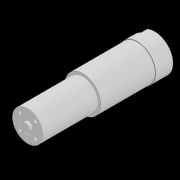
# Autodesk Inventor part: ShoulderServo
Saved by Autodesk Inventor 2020 (Build 240168000, 168)
## iProperties
Created: 2021-01-27
Part Number: ShoulderServo
Material: Generic
Document SubType Name: Modeling
Designer: valer
Density: 1 g/cm^3
Appearance: Default
Author: valer
Autodesk Inventor part; units mm, degrees
ref_plane "YZ Plane" through (0, 0, 0) normal (1, 0, 0) x (0, 1, 0)
ref_plane "XZ Plane" through (0, 0, 0) normal (0, 1, 0) x (-1, 0, 0)
ref_plane "XY Plane" through (0, 0, 0) normal (0, 0, 1) x (1, 0, 0)
sketch "Base" plane through (0, 0, 0) normal (0, 0, 1) x (1, 0, 0)
  circle A0 centre (0, 0) radius 18.75
  dimension "d0" = 37.5
  constraints: 1 centre point, 1 coincident
  measures "d0" diameter of A0
extrude "BaseFeature" add sketch "Base" along normal blind 57
sketch "Sketch2" plane through (0, 0, 0) normal (0, 0, -1) x (-1, 0, 0)
  circle A0 centre (0, 0) radius 18.75 projected
  circle A1 centre (0, 0) radius 19.25
  dimension "d3" = 0.5
  constraints: 1 centre point, 1 coincident
  measures "d3" radial gap between concentric circles of A1 A0
extrude "BottomFeature" add sketch "Sketch2" along normal blind 18.2 contours A0 | A1
sketch "Panel" plane through (0, 0, -18.2) normal (0, 0, -1) x (-1, 0, 0)
  circle A0 centre (0, 0) radius 19.25 projected
  line L0 (7.75, 17.621) -> (7.75, -17.621)
  circle A1 centre (0, 0) radius 18.75 construction
  line L1 (0, 0) -> (-19.25, 0) construction
  circle A2 centre (0, 0) radius 19.25 projected
  line L2 (7.75, 17.621) -> (19.25, 17.621)
  line L3 (19.25, 17.621) -> (19.25, -17.621)
  line L4 (19.25, -17.621) -> (7.75, -17.621)
  line L5 (7.75, -17.621) -> (7.75, 17.621)
  dimension "d6" = 27
  constraints: 12 end point, 3 point on circle, 2 horizontal, 2 parallel, 1 perpendicular, 1 point on line, 1 tangent, 1 vertical
  measures "d6" distance from line of L1.end L0
extrude "PanelFeature" cut sketch "Panel" against normal blind 6.5 contours A0 L0 picked at (11.5833, 0)
sketch "Gearbox" plane through (0, 0, 57) normal (0, 0, 1) x (1, 0, 0)
  circle A0 centre (0, 0) radius 16
  dimension "d9" = 32
  constraints: 1 centre point, 1 coincident
  measures "d9" diameter of A0
extrude "GearboxFeature" add sketch "Gearbox" along normal blind 57.8
sketch "Shaft" plane through (0, 0, 114.8) normal (0, 0, 1) x (1, 0, 0)
  circle A0 centre (0, 0) radius 18.75 projected
  circle A1 centre (0, 0) radius 8
  dimension "d12" = 16
  constraints: 1 centre point, 1 coincident
  measures "d12" diameter of A1
extrude "ShaftFeature" cut sketch "Shaft" against normal blind 1 contours A1
sketch "MountHoles" plane through (0, 0, 114.8) normal (0, 0, 1) x (1, 0, 0)
  line L0 (0, 0) -> (-19.25, 0) construction
  line L1 (0, 0) -> (0, 19.25) construction
  circle A0 centre (0, 0) radius 19.25 construction
  line L2 (-8, -8) -> (8, -8) construction
  line L3 (8, -8) -> (8, 8) construction
  line L4 (8, 8) -> (-8, 8) construction
  line L5 (-8, 8) -> (-8, -8) construction
  circle A1 centre (-8, -8) radius 1.65
  circle A2 centre (-8, 8) radius 1.65
  circle A3 centre (8, 8) radius 1.65
  circle A4 centre (8, -8) radius 1.65
  point P0 (-8, 0)
  point P1 (0, 8)
  dimension "d16" = 16
  dimension "d17" = 3.3
  constraints: 12 end point, 4 centre point, 4 coincident, 3 equal radius, 2 horizontal, 2 midpoint, 2 parallel, 2 perpendicular, 2 point on circle, 2 point on line, 1 vertical
  measures "d16" distance of L4.end L2.start
  measures "d17" diameter of A1
extrude "MountHolesFeature" cut sketch "MountHoles" against normal blind 10
sketch "ShaftBase" plane through (0, 0, 114.8) normal (0, 0, 1) x (1, 0, 0)
  circle A0 centre (0, 0) radius 4
  dimension "d22" = 8
  constraints: 1 centre point, 1 coincident
  measures "d22" diameter of A0
extrude "ShaftBaseFeature" add sketch "ShaftBase" along normal mid plane 5
body "Solid1"
